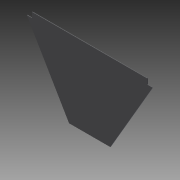
# Autodesk Inventor part: electrical board back
Saved by Autodesk Inventor 2012 (Build 160160000, 160)
## iProperties
Created: 2011-10-06
Part Number: electrical board back
Material: ABS Plastic
Document SubType Name: Modeling
Designer: Antonella
Mass: 534.136 g
Surface Area: 3227.61 cm^2
Volume: 503.902 cm^3
Density: 1.06 g/cm^3
Author: Antonella
Autodesk Inventor part; units mm, degrees
ref_plane "YZ Plane" through (0, 0, 0) normal (1, 0, 0) x (0, 1, 0)
ref_plane "XZ Plane" through (0, 0, 0) normal (0, 1, 0) x (-1, 0, 0)
ref_plane "XY Plane" through (0, 0, 0) normal (0, 0, 1) x (1, 0, 0)
sketch "Sketch1" plane through (0, 0, 0) normal (0, 0, 1) x (1, 0, 0)
  line L0 (-420.0525, 0) -> (420.0525, 0) projected
  line L1 (0, -420.37) -> (0, 99.695) projected
  line L2 (-274.6375, 25.4) -> (274.6375, 25.4)
  line L3 (-98.425, -346.075) -> (98.425, -346.075)
  line L4 (-274.6375, 25.4) -> (-274.6375, 0)
  line L5 (-274.6375, 0) -> (-300.0375, 0)
  line L6 (-300.0375, 0) -> (-98.425, -346.075)
  line L7 (274.6375, 25.4) -> (274.6375, 0)
  line L8 (274.6375, 0) -> (300.0375, 0)
  line L9 (300.0375, 0) -> (98.425, -346.075)
  point P0 (0, 0)
  point P1 (0, 25.4)
  point P2 (0, -346.075)
  dimension "d0" = 196.85
  dimension "d2" = 371.475
  dimension "d3" = 25.4
  dimension "d6" = 600.075
  constraints: 16 end point, 7 perpendicular, 2 midpoint, 2 point on line, 2 vertical alignment, 1 parallel
  measures "d0" distance of L3.start L3.end
  measures "d2" distance between parallel lines of L2 L3
  measures "d3" distance of L2.start L4.end
  measures "d6" distance of L5.end L8.end
extrude "Extrusion1" add sketch "Sketch1" along normal mid plane 3.175
body "Solid1"
